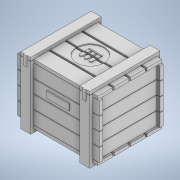
# Autodesk Inventor part: Ammo-Item-Large
Saved by Autodesk Inventor 2020 (Build 240168000, 168)
## iProperties
Created: 2019-10-06
Part Number: Ammo-Item-Large
Material: Generic
Document SubType Name: Modeling
Designer: Victor
Density: 1 g/cm^3
Appearance: Default
Author: Victor
Autodesk Inventor part; units mm, degrees
ref_plane "YZ Plane" through (0, 0, 0) normal (1, 0, 0) x (0, 1, 0)
ref_plane "XZ Plane" through (0, 0, 0) normal (0, 1, 0) x (-1, 0, 0)
ref_plane "XY Plane" through (0, 0, 0) normal (0, 0, 1) x (1, 0, 0)
sketch "Sketch1" plane through (0, 0, 0) normal (0, 0, 1) x (1, 0, 0)
  line L0 (0, 0.25) -> (12.5, 0.25)
  line L1 (12.5, 0.25) -> (12.5, 4.25)
  line L2 (12.5, 4.25) -> (0, 4.25)
  line L3 (0, 4.25) -> (-12.5, 4.25)
  line L4 (-12.5, 4.25) -> (-12.5, 0.25)
  line L5 (-12.5, 0.25) -> (0, 0.25)
  dimension "d5" = 4
  dimension "d6" = 12.5
  dimension "d7" = 12.5
  dimension "d8" = 12.5
  dimension "d9" = 12.5
  dimension "d10" = 25
  constraints: 12 end point, 2 parallel, 1 horizontal, 1 perpendicular
  measures "d5" distance of L1.end L0.end
  measures "d6" distance of L3.end L2.end
  measures "d7" distance of L0.start L4.end
  measures "d8" distance of L1.end L2.end
  measures "d9" distance of L0.start L0.end
  measures "d10" horizontal distance of L4.end L1.end
extrude "Extrusion2" add sketch "Sketch1" against normal blind 1
pattern_linear "Rectangular Pattern1" count 4 spacing 4.125 along (0, -1, 0) of "Extrusion2"
sketch "Sketch2" plane through (0, 0, -1) normal (0, 0, -1) x (-1, 0, 0)
  line L0 (12.5, 4.25) -> (-12.5, 4.25) projected
  line L1 (10.5, 4.25) -> (11.5, 4.25)
  line L2 (11.5, 4.25) -> (11.5, 0.25)
  line L3 (11.5, 0.25) -> (10.5, 0.25)
  line L4 (10.5, 0.25) -> (10.5, 4.25)
  point P0 (0, 0)
  dimension "d16" = 1
  constraints: 8 end point, 2 parallel, 1 perpendicular, 1 point on line
  measures "d16" distance of L1.start L1.end
extrude "Extrusion3" add sketch "Sketch2" along normal blind 17.5
pattern_linear "Rectangular Pattern2" count 4 spacing 4.125 along (0, -1, 0) of "Extrusion3"
pattern_linear "Rectangular Pattern3" count 2 spacing 22 along (1, 0, 0) of "Extrusion3", "Rectangular Pattern2"
pattern_linear "Rectangular Pattern4" count 2 spacing 18.5 along (0, 0, -1) of "Extrusion2", "Rectangular Pattern1"
sketch "Sketch3" plane through (0, 0, 0) normal (0, 0, 1) x (1, 0, 0)
  line L0 (-10.5, 5.25) -> (-10.5, -13.125)
  line L1 (-10.5, -13.125) -> (-7.5, -13.125)
  line L2 (-7.5, -13.125) -> (-7.5, 5.25)
  line L3 (-7.5, 5.25) -> (-10.5, 5.25)
  line L4 (10.5, 5.25) -> (10.5, -13.125)
  line L5 (10.5, -13.125) -> (7.5, -13.125)
  line L6 (7.5, -13.125) -> (7.5, 5.25)
  line L7 (7.5, 5.25) -> (10.5, 5.25)
  point P0 (0, 0)
  dimension "d28" = 18.375
  dimension "d29" = 3
  dimension "d30" = 3
  constraints: 16 end point, 4 parallel, 3 perpendicular, 2 point on line, 1 vertical
  measures "d28" distance of L0.start L0.end
  measures "d29" distance of L1.end L0.end
  measures "d30" distance of L4.end L5.end
extrude "Extrusion4" add sketch "Sketch3" along normal blind 1
pattern_linear "Rectangular Pattern5" count 2 spacing 20.5 along (0, 0, -1) of "Extrusion4"
sketch "Sketch4" plane through (7.5, 5.25, 0) normal (0, 1, 0) x (1, 0, 0)
  line L0 (3, -1) -> (0, -1) projected
  line L1 (3, 20.5) -> (0, 20.5) projected
  line L2 (3, -1) -> (3, 20.5)
  line L3 (3, 20.5) -> (0, 20.5)
  line L4 (0, 20.5) -> (0, -1)
  line L5 (0, -1) -> (3, -1)
  line L6 (-18, -1) -> (-15, -1) projected
  line L7 (-18, -1) -> (-15, -1)
  line L8 (-15, -1) -> (-15, 20.5)
  line L9 (-15, 20.5) -> (-18, 20.5)
  line L10 (-18, 20.5) -> (-18, -1)
  point P0 (-7.5, 0)
  constraints: 16 end point, 5 equal length, 2 perpendicular, 1 vertical
extrude "Extrusion5" add sketch "Sketch4" along normal blind 1
sketch "Sketch5" plane through (7.5, 5.25, 0) normal (0, -1, 0) x (1, 0, 0)
  line L0 (-20, -19.5) -> (-18, -19.5) projected
  line L1 (3, -19.5) -> (5, -19.5) projected
  line L2 (-19.5, -19.5) -> (4, -19.5)
  line L3 (4, -19.5) -> (4, -15)
  line L4 (4, -15) -> (-19.5, -15)
  line L5 (-19.5, -15) -> (-19.5, -19.5)
  point P0 (-7.5, 0)
  dimension "d38" = 4.5
  constraints: 8 end point, 2 parallel, 1 midpoint, 1 perpendicular, 1 point on line
  measures "d38" distance of L3.end L2.end
extrude "Extrusion6" add sketch "Sketch5" along normal blind 0.95
pattern_linear "Rectangular Pattern6" count 4 spacing 5 along (0, 0, 1) of "Extrusion6"
sketch "Sketch6" plane through (10.5, -13.125, -20.5) normal (0, 0, -1) x (-1, 0, 0)
  line L0 (-1, 18.375) -> (0, 18.375) projected
  line L1 (0, 18.375) -> (21, 18.375)
  line L2 (21, 0) -> (21, 19.375) projected
  line L3 (21, 18.275) -> (0, 18.275)
  line L4 (0, 18.275) -> (-1, 18.275)
  line L5 (22.5, 18.375) -> (21, 18.375) projected
  line L6 (21, 18.375) -> (21, 18.275)
  line L7 (0, 18.375) -> (3, 18.375) projected
  line L8 (0, 18.375) -> (0, 18.275)
  line L9 (0, 17.425) -> (0, 18.375) projected
  point P0 (10.5, 13.125)
  dimension "d45" = 0.1
  constraints: 10 end point, 1 collinear, 1 horizontal, 1 vertical, 1 other
  measures "d45" distance between parallel lines of L1 L3
extrude "Extrusion7" cut sketch "Sketch6" against normal blind 1
sketch "Sketch7" plane through (10.5, 6.25, -20.5) normal (0, 0, -1) x (-1, 0, 0)
  line L0 (0, 0) -> (3, 0) projected
  line L1 (1, 0) -> (2, 0)
  line L2 (2, 0) -> (2, -3)
  line L3 (2, -3) -> (1, -3)
  line L4 (1, -3) -> (1, 0)
  line L5 (18, 0) -> (21, 0) projected
  line L6 (19, 0) -> (20, 0)
  line L7 (20, 0) -> (20, -3)
  line L8 (20, -3) -> (19, -3)
  line L9 (19, -3) -> (19, 0)
  point P0 (10.5, -6.25)
  dimension "d48" = 1
  dimension "d49" = 3
  dimension "d50" = 1
  constraints: 16 end point, 4 parallel, 4 point on line, 2 perpendicular
  measures "d48" distance of L1.start L1.end
  measures "d49" distance of L1.end L2.end
  measures "d50" distance of L6.start L6.end
extrude "Extrusion8" add sketch "Sketch7" along normal blind 0.25
pattern_linear "Rectangular Pattern7" count 2 spacing 19.375 along (0, -1, 0) of "Extrusion5"
pattern_linear "Rectangular Pattern8" count 2 spacing 17.425 along (0, -1, 0) of "Extrusion6", "Rectangular Pattern6"
sketch "Sketch9" plane through (-7.5, 5.25, -5) normal (0, 1, 0) x (1, 0, 0)
  circle A0 centre (7.5, 4.75) radius 4.1875
  line L0 (7, 3.5) -> (7, 6)
  line L1 (7, 6) -> (8, 6)
  line L2 (8, 6) -> (8, 3.5)
  line L3 (8, 3.5) -> (7, 3.5)
  line L4 (7, 3.5) -> (8, 6) construction
  line L5 (7, 6) -> (8, 3.5) construction
  arc A1 (8, 6) -> (7, 6) centre (7.5, 6) ccw
  line L6 (8.5, 3.5) -> (8.5, 6)
  line L7 (8.5, 6) -> (9.5, 6)
  line L8 (9.5, 6) -> (9.5, 3.5)
  line L9 (9.5, 3.5) -> (8.5, 3.5)
  line L10 (8.5, 3.5) -> (9.5, 6) construction
  line L11 (8.5, 6) -> (9.5, 3.5) construction
  arc A2 (9.5, 6) -> (8.5, 6) centre (9, 6) ccw
  line L12 (5.5, 3.5) -> (5.5, 6)
  line L13 (5.5, 6) -> (6.5, 6)
  line L14 (6.5, 6) -> (6.5, 3.5)
  line L15 (6.5, 3.5) -> (5.5, 3.5)
  line L16 (5.5, 3.5) -> (6.5, 6) construction
  line L17 (5.5, 6) -> (6.5, 3.5) construction
  arc A3 (6.5, 6) -> (5.5, 6) centre (6, 6) ccw
  line L18 (7, 3.5) -> (7, 6)
  line L19 (7, 6) -> (8, 6)
  line L20 (8, 6) -> (8, 3.5)
  line L21 (8, 3.5) -> (7, 3.5)
  line L22 (7, 3.5) -> (8, 6) construction
  line L23 (7, 6) -> (8, 3.5) construction
  arc A4 (8, 6) -> (7, 6) centre (7.5, 6) ccw
  line L24 (9.5, 3) -> (5.5, 3)
  line L25 (5.5, 3) -> (5.5, 3.35)
  line L26 (5.5, 3.35) -> (9.5, 3.35)
  line L27 (9.5, 3.35) -> (9.5, 3)
  point P0 (7.5, -5)
  point P1 (7.5, -0.125)
  point P2 (9, 4.75)
  point P3 (6, 4.75)
  dimension "d77" = 2.5
  dimension "d78" = 1
  dimension "d79" = 1.5
  dimension "d80" = 1.5
  dimension "d81" = 9.75
  constraints: 56 end point, 8 midpoint, 8 point on circle, 5 centre point, 4 parallel, 3 horizontal, 2 collinear, 2 perpendicular, 2 tangent, 1 vertical, 37 other
  measures "d77" distance of L0.start L0.end
  measures "d78" distance of L0.end L2.start
  measures "d79" distance of A0.centre point (9, 4.75)
  measures "d80" distance of A0.centre point (6, 4.75)
  measures "d81" distance of A0.centre point (7.5, -5)
extrude "Extrusion10" cut sketch "Sketch9" against normal blind 0.25
sketch "Sketch10" plane through (7.5, 0.125, -19.5) normal (0, 0, -1) x (-1, 0, 0)
  line L0 (4, -1) -> (11, -1)
  line L1 (11, -1) -> (11, -3)
  line L2 (11, -3) -> (4, -3)
  line L3 (4, -3) -> (4, -1)
  point P0 (7.5, -0.125)
  dimension "d84" = 7
  dimension "d85" = 2
  constraints: 8 end point, 2 parallel, 1 horizontal, 1 perpendicular
  measures "d84" distance of L1.end L2.end
  measures "d85" distance of L0.end L1.end
extrude "Extrusion11" add sketch "Sketch10" along normal blind 0.25
body "Solid2"
